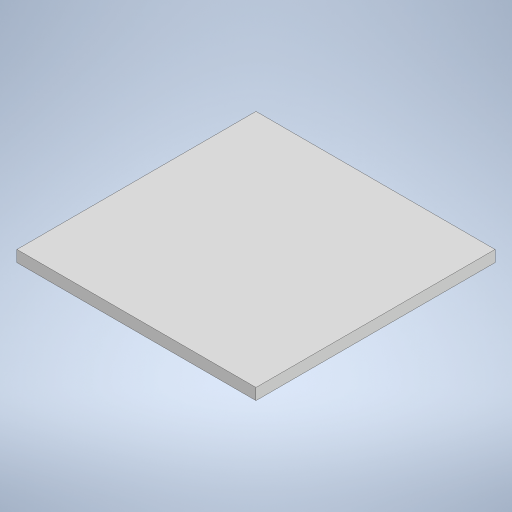
# Autodesk Inventor part: mein1
Saved by Autodesk Inventor 2023 (Build 270158000, 158)
## iProperties
Created: 2022-10-24
Part Number: mein1
Material: 一般
Document SubType Name: Modeling
Designer: ellie
Density: 1 g/cm^3
Appearance: 既定
Author: ellie
Autodesk Inventor part; units mm, degrees
ref_plane "YZ Plane" through (0, 0, 0) normal (1, 0, 0) x (0, 1, 0)
ref_plane "XZ Plane" through (0, 0, 0) normal (0, 1, 0) x (-1, 0, 0)
ref_plane "XY Plane" through (0, 0, 0) normal (0, 0, 1) x (1, 0, 0)
sketch "スケッチ1" plane through (0, 0, 0) normal (0, 1, 0) x (-1, 0, 0)
  line L0 (21, 21) -> (-21, 21)
  line L1 (-21, 21) -> (-21, -21)
  line L2 (-21, -21) -> (21, -21)
  line L3 (21, -21) -> (21, 21)
  line L4 (21, 21) -> (-21, -21) construction
  line L5 (-21, 21) -> (21, -21) construction
  point P0 (0, 0)
  dimension "d0" = 42
  dimension "d1" = 42
  constraints: 12 end point, 2 midpoint, 2 parallel, 1 horizontal, 1 perpendicular
  measures "d0" distance of L0.start L0.end
  measures "d1" distance of L0.end L1.end
extrude "押し出し1" add sketch "スケッチ1" along normal blind 2
